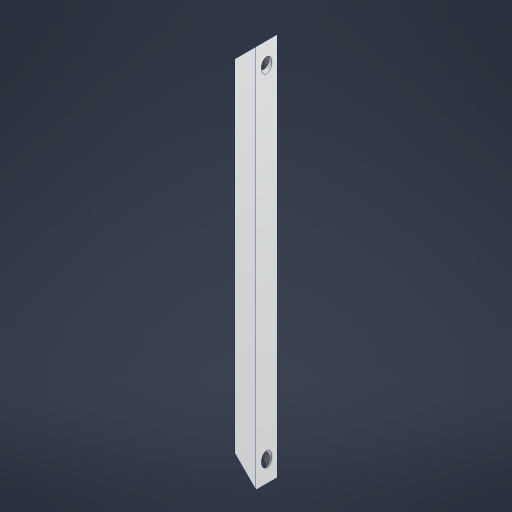
# Autodesk Inventor part: STRU_010_BilletCrossbar_17.7in_Angled
Saved by Autodesk Inventor 2024.2 (Build 282272000, 272)
## iProperties
Created: 2024-07-24
Part Number: STRU_010_BilletCrossbar_17.7in_Angled
Material: Aluminum 6061
Document SubType Name: Modeling
Designer: Bryan
Density: 2.7 g/cm^3
Appearance: Aluminum - Flat
Author: Bryan
Autodesk Inventor part; units mm, degrees
ref_plane "YZ Plane" through (0, 0, 0) normal (1, 0, 0) x (0, 1, 0)
ref_plane "XZ Plane" through (0, 0, 0) normal (0, 1, 0) x (-1, 0, 0)
ref_plane "XY Plane" through (0, 0, 0) normal (0, 0, 1) x (1, 0, 0)
sketch "Sketch1" plane through (0, 0, 0) normal (0, 1, 0) x (-1, 0, 0)
  line L0 (-12.7, -12.7) -> (12.7, -12.7)
  line L1 (12.7, -12.7) -> (12.7, 12.7)
  line L2 (12.7, 12.7) -> (-12.7, 12.7)
  line L3 (-12.7, 12.7) -> (-12.7, -12.7)
  line L4 (-12.7, -12.7) -> (12.7, 12.7) construction
  line L5 (12.7, -12.7) -> (-12.7, 12.7) construction
  line L6 (9.525, 9.525) -> (9.525, -9.525)
  line L7 (9.525, -9.525) -> (-9.525, -9.525)
  line L8 (-9.525, -9.525) -> (-9.525, 9.525)
  line L9 (-9.525, 9.525) -> (9.525, 9.525)
  point P0 (0, 0)
  dimension "d0" = 25.4
  dimension "d1" = 25.4
  dimension "d2" = 3.175
  constraints: 20 end point, 4 parallel, 2 midpoint, 2 perpendicular, 1 horizontal, 3 other
  measures "d0" distance of L2.end L1.end
  measures "d1" distance of L1.end L0.end
  measures "d2" distance between parallel lines of L1 L6
extrude "Extrusion1" add sketch "Sketch1" along normal blind 458.597
sketch "Sketch2" plane through (12.7, 0, -12.7) normal (0, 0, -1) x (-1, 0, 0)
  line L0 (0, 0) -> (25.4, 25.4)
  line L1 (25.4, 0) -> (25.4, 458.597) projected
  line L2 (0, 0) -> (25.4, 0) projected
  line L3 (25.4, 0) -> (25.4, 458.597) projected
  line L4 (0, 458.597) -> (25.4, 458.597) projected
  line L5 (0, 0) -> (0, 458.597) projected
  line L6 (0, 458.597) -> (25.4, 433.197)
  point P0 (12.7, 0)
  dimension "d5" = 25.4
  dimension "d6" = 25.4
  constraints: 4 end point, 2 point on line
  measures "d5" distance of L1.start L0.end
  measures "d6" distance of L1.end L6.end
extrude "Extrusion2" cut sketch "Sketch2" against normal blind 451.1802 contours L0 L1 L2 | L4 L1 L6
sketch "Sketch3" plane through (12.7, 0, 12.7) normal (-0.7071068, -0.7071068, 0) x (-0.7071068, 0.7071068, 0)
  line L0 (35.921, 0) -> (0, 0) projected
  line L1 (35.921, 25.4) -> (35.921, 0) projected
  line L2 (0, 25.4) -> (35.921, 25.4) projected
  line L3 (0, 0) -> (0, 25.4) projected
  line L4 (4.4901, 3.175) -> (31.4309, 3.175) projected
  line L5 (4.4901, 22.225) -> (4.4901, 3.175) projected
  line L6 (31.4309, 22.225) -> (4.4901, 22.225) projected
  line L7 (31.4309, 3.175) -> (31.4309, 22.225) projected
  line L8 (35.921, 0) -> (324.277, 0) projected
  line L9 (35.921, 0) -> (0, 25.4)
  line L10 (35.921, 25.4) -> (0, 0)
  circle A0 centre (17.9605, 12.7) radius 6.35
  point P0 (8.9803, 12.7)
  dimension "d9" = 12.7
  constraints: 4 end point, 1 centre point, 1 midpoint
  measures "d9" diameter of A0
extrude "Extrusion3" cut sketch "Sketch3" against normal through all contours A0 L10 L9 | L9 L10 A0 | A0 L9 L10 | L10 L9 A0
sketch "Sketch4" plane through (12.7, 458.597, -12.7) normal (-0.7071068, 0.7071068, 0) x (-0.7071068, -0.7071068, 0)
  line L0 (0, 25.4) -> (35.921, 25.4) construction
  line L1 (0, 25.4) -> (0, 0) construction
  line L2 (35.921, 0) -> (0, 0) construction
  line L3 (35.921, 25.4) -> (35.921, 0) construction
  line L4 (31.4309, 22.225) -> (4.4901, 22.225) construction
  line L5 (31.4309, 3.175) -> (31.4309, 22.225) construction
  line L6 (4.4901, 3.175) -> (31.4309, 3.175) construction
  line L7 (4.4901, 22.225) -> (4.4901, 3.175) construction
  line L8 (0, 0) -> (35.921, 25.4) construction
  line L9 (35.921, 0) -> (0, 25.4) construction
  circle A0 centre (17.9605, 12.7) radius 6.35
  point P0 (333.2573, 12.7)
  dimension "d12" = 12.7
  constraints: 4 end point, 1 centre point, 1 midpoint
  measures "d12" diameter of A0
extrude "Extrusion4" cut sketch "Sketch4" against normal through all
body "Solid1"
